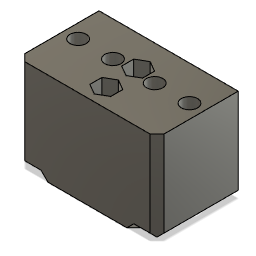
Hanger__Ceiling__Interchange (Autodesk Fusion 360 design; units mm, degrees)
Autodesk Fusion 360 part; units mm, degrees
sketch "Sketch1" plane through (0, 0, 0) normal (0, 1, 0) x (1, 0, 0)
  line L0 (0, 0) -> (60, 0)
  line L1 (60, 0) -> (60, -40)
  line L2 (60, -40) -> (0, -40)
  line L3 (0, -40) -> (0, 0)
  dimension "d1" = 60
  dimension "d2" = 40
  constraint horizontal L0
  constraint vertical L1
  constraint horizontal L2
  constraint vertical L3
  constraint coincident L0.start L3.end
  measures "d1" distance of L0.start L0.end
  measures "d2" distance of L0.start L2.end
extrude "Extrude1" add sketch "Sketch1" along normal blind 25
sketch "Sketch2" plane through (0, 25, 0) normal (0, 1, 0) x (-1, 0, 0)
  line L0 (0, 40) -> (-60, 40)
  line L1 (-60, 40) -> (-60, 0)
  line L2 (-60, 0) -> (0, 0)
  line L3 (0, 0) -> (0, 40)
  line L4 (-30, 0) -> (-30, 20)
  line L5 (-30, 20) -> (-39, 20)
  line L6 (-30, 20) -> (-21, 20)
  line L7 (-21, 20) -> (-6, 20)
  line L8 (-39, 20) -> (-54, 20)
  circle A0 centre (-21, 20) radius 3.5
  circle A1 centre (-39, 20) radius 3.5
  circle A2 centre (-54, 20) radius 3.5
  circle A3 centre (-6, 20) radius 3.5
  dimension "d5" = 20
  dimension "d6" = 9
  dimension "d7" = 9
  dimension "d8" = 15
  dimension "d9" = 15
  dimension "d10" = 7
  dimension "d11" = 7
  dimension "d12" = 7
  dimension "d13" = 7
  constraint midpoint L2 L4.start
  constraint perpendicular L0 L4
  constraint perpendicular L4 L5
  constraint perpendicular L4 L6
  constraint parallel L6 L7
  constraint perpendicular L4 L8
  constraint coincident L6.end L7.start
  constraint coincident L5.end L8.start
  constraint coincident L8.end A2.centre
  constraint coincident L7.end A3.centre
  measures "d5" distance of L4.start L4.end
  measures "d6" distance of L4.end L5.end
  measures "d7" distance of L4.end L6.end
  measures "d8" distance of L6.end L7.end
  measures "d9" distance of L5.end L8.end
  measures "d10" diameter of A0
  measures "d11" diameter of A1
  measures "d12" diameter of A2
  measures "d13" diameter of A3
extrude "Extrude2" cut sketch "Sketch2" against normal blind 25 contours L5 L8 A1 | L5 L8 A1 | L6 L7 A0 | L6 L7 A0 | A2 | A3
sketch "Sketch3" plane through (0, 0, 0) normal (0, -1, 0) x (1, 0, 0)
  circle A0 centre (21, 20) radius 3.5
  circle A1 centre (39, 20) radius 3.5
  circle A2 centre (6, 20) radius 3.5
  circle A3 centre (54, 20) radius 3.5
  line L0 (60, 40) -> (0, 40)
  line L1 (0, 40) -> (0, 0)
  line L2 (0, 0) -> (60, 0)
  line L3 (60, 0) -> (60, 40)
  circle A4 centre (6, 20) radius 6.5
  circle A5 centre (21, 20) radius 6.5
  circle A6 centre (39, 20) radius 6.5
  circle A7 centre (54, 20) radius 6.5
  dimension "d16" = 13
  dimension "d17" = 13
  dimension "d18" = 13
  dimension "d19" = 13
  constraint concentric A2 A4
  constraint concentric A0 A5
  constraint concentric A1 A6
  constraint concentric A3 A7
  measures "d16" diameter of A4
  measures "d17" diameter of A5
  measures "d18" diameter of A6
  measures "d19" diameter of A7
extrude "Extrude3" cut sketch "Sketch3" against normal blind 2 contours L3 A7 | L1 A4 | A5 | A6 picked at (59.1667, 20) picked at (0.8333, 20)
extrude "Extrude4" cut 4 faces at (0.8333, 2, 20) (26.4628, 2, 19.5032) (44.4758, 2, 19.6771) (59.1667, 2, 20) along direction (0, 1, 0) blind 13
sketch "Sketch4" plane through (0, 25, 0) normal (0, 1, 0) x (-1, 0, 0)
  circle A0 centre (-21, 20) radius 3.5
  circle A1 centre (-39, 20) radius 3.5
  circle A2 centre (-6, 20) radius 3.5
  circle A3 centre (-54, 20) radius 3.5
  line L0 (0, 40) -> (-60, 40)
  line L1 (-60, 40) -> (-60, 0)
  line L2 (-60, 0) -> (0, 0)
  line L3 (0, 0) -> (0, 40)
  line L4 (-30, 40) -> (-30, 0)
  line L5 (-30, 20) -> (-30, 26.85)
  line L6 (-30, 26.85) -> (-30, 13.15)
  circle A4 centre (-30, 13.15) radius 2
  circle A5 centre (-30, 26.85) radius 2
  dimension "d24" = 6.85
  dimension "d25" = 13.7
  dimension "d26" = 4
  dimension "d27" = 4
  constraint midpoint L0 L4.start
  constraint midpoint L2 L4.end
  constraint midpoint L4 L5.start
  constraint parallel L4 L5
  constraint parallel L4 L6
  constraint coincident L6.end A4.centre
  constraint coincident L5.end L6.start
  measures "d24" distance of L5.start L5.end
  measures "d25" distance of L5.end L6.end
  measures "d26" diameter of A4
  measures "d27" diameter of A5
sketch "Sketch5" plane through (0, 25, 0) normal (0, 1, 0) x (-1, 0, 0)
  circle A0 centre (-21, 20) radius 3.5
  circle A1 centre (-39, 20) radius 3.5
  circle A2 centre (-6, 20) radius 3.5
  circle A3 centre (-54, 20) radius 3.5
  line L0 (0, 40) -> (-60, 40)
  line L1 (-60, 40) -> (-60, 0)
  line L2 (-60, 0) -> (0, 0)
  line L3 (0, 0) -> (0, 40)
  line L4 (-34.5, 24.2519) -> (-30, 21.6538)
  line L5 (-30, 21.6538) -> (-25.5, 24.2519)
  line L6 (-25.5, 24.2519) -> (-25.5, 29.4481)
  line L7 (-25.5, 29.4481) -> (-30, 32.0462)
  line L8 (-30, 32.0462) -> (-34.5, 29.4481)
  line L9 (-34.5, 29.4481) -> (-34.5, 24.2519)
  line L10 (-34.5, 10.5519) -> (-30, 7.9538)
  line L11 (-30, 7.9538) -> (-25.5, 10.5519)
  line L12 (-25.5, 10.5519) -> (-25.5, 15.7481)
  line L13 (-25.5, 15.7481) -> (-30, 18.3462)
  line L14 (-30, 18.3462) -> (-34.5, 15.7481)
  line L15 (-34.5, 15.7481) -> (-34.5, 10.5519)
  point P0 (-30, 26.85)
  point P1 (-30, 13.15)
  dimension "d30" = 4.5
  dimension "d31" = 4.5
  measures "d30" distance of P0 L9
  measures "d31" distance of P1 L15
sketch "Sketch6" plane through (0, 0, 0) normal (0, -1, 0) x (1, 0, 0)
  arc A0 (60, 22.5) -> (60, 17.5) centre (54, 20) ccw
  line L0 (60, 22.5) -> (60, 40)
  line L1 (60, 40) -> (0, 40)
  line L2 (0, 40) -> (0, 22.5)
  arc A1 (0, 17.5) -> (0, 22.5) centre (6, 20) ccw
  line L3 (0, 17.5) -> (0, 0)
  line L4 (0, 0) -> (60, 0)
  line L5 (60, 0) -> (60, 17.5)
  circle A2 centre (21, 20) radius 6.5
  circle A3 centre (39, 20) radius 6.5
  circle A4 centre (6, 20) radius 5
  circle A5 centre (21, 20) radius 5
  circle A6 centre (54, 20) radius 5
  circle A7 centre (39, 20) radius 5
  circle A8 centre (6, 20) radius 6.5
  circle A9 centre (54, 20) radius 6.5
  circle A10 centre (39, 20) radius 6.5
  circle A11 centre (21, 20) radius 6.5
  dimension "d32" = 10
  dimension "d33" = 10
  dimension "d34" = 10
  dimension "d35" = 10
  constraint concentric A1 A4
  constraint concentric A2 A5
  constraint concentric A0 A6
  constraint concentric A3 A7
  constraint concentric A4 A8
  constraint concentric A6 A9
  constraint concentric A7 A10
  constraint concentric A5 A11
  measures "d32" diameter of A4
  measures "d33" diameter of A5
  measures "d34" diameter of A6
  measures "d35" diameter of A7
extrude "Extrude6" add sketch "Sketch6" against normal blind 15 contours A0 A9 | A1 A8 | A2 A11 | A3 A10
sketch "Sketch7" plane through (0, 25, 0) normal (0, 1, 0) x (-1, 0, 0)
  circle A0 centre (-21, 20) radius 3.5
  circle A1 centre (-39, 20) radius 3.5
  circle A2 centre (-6, 20) radius 3.5
  circle A3 centre (-54, 20) radius 3.5
  line L0 (0, 40) -> (-60, 40)
  line L1 (-60, 40) -> (-60, 0)
  line L2 (-60, 0) -> (0, 0)
  line L3 (0, 0) -> (0, 40)
  line L4 (-60, 40) -> (0, 40)
  line L5 (0, 40) -> (0, 0)
  line L6 (0, 0) -> (-60, 0)
  line L7 (-60, 0) -> (-60, 40)
  line L8 (-63.5098, 43.7878) -> (2.9374, 43.7878)
  line L9 (2.9374, 43.7878) -> (2.9374, -3.4155)
  line L10 (2.9374, -3.4155) -> (-63.5098, -3.4155)
  line L11 (-63.5098, -3.4155) -> (-63.5098, 43.7878)
  constraint horizontal L4
  constraint vertical L5
  constraint horizontal L6
  constraint vertical L7
  constraint coincident L2.end L3.start
  constraint coincident L0.end L1.start
  constraint horizontal L8
  constraint vertical L9
  constraint horizontal L10
  constraint vertical L11
extrude "Extrude8" cut sketch "Sketch7" against normal blind 41 contours L8 L9 L10 L11
sketch "Sketch8" plane through (0, 0, 0) normal (-1, 0, 0) x (0, 0, 1)
  line L0 (0, 0) -> (40, 0)
  line L1 (40, 0) -> (40, 25)
  line L2 (40, 25) -> (0, 25)
  line L3 (0, 25) -> (0, 0)
  line L4 (40, 0) -> (37, 0)
  line L5 (40, 0) -> (40, 3)
  line L6 (40, 3) -> (37, 0)
  dimension "d42" = 3
  dimension "d43" = 3
  constraint coincident L0.end L1.start
  constraint perpendicular L1 L4
  constraint perpendicular L0 L5
  measures "d42" distance of L0.end L4.end
  measures "d43" distance of L0.end L5.end
extrude "Extrude9" cut sketch "Sketch8" against normal blind 10 contours L0 L1 L4 L5 L6
extrude "Extrude10" cut 1 faces at (10, 1, 39) along direction (-1, 0, 0) blind -40 and the other way blind 50
sketch "Sketch9" plane through (0, 25, 0) normal (0, 1, 0) x (-1, 0, 0)
  circle A0 centre (-21, 20) radius 3.5
  circle A1 centre (-39, 20) radius 3.5
  circle A2 centre (-6, 20) radius 3.5
  circle A3 centre (-54, 20) radius 3.5
  line L0 (0, 40) -> (-60, 40)
  line L1 (-60, 40) -> (-60, 0)
  line L2 (-60, 0) -> (0, 0)
  line L3 (0, 0) -> (0, 40)
  line L4 (-30, 40) -> (-30, 31.85)
  circle A4 centre (-30, 31.85) radius 2
  line L5 (-30, 31.85) -> (-30, 18.15)
  circle A5 centre (-30, 18.15) radius 2
  dimension "d50" = 8.15
  dimension "d51" = 4
  dimension "d52" = 13.7
  dimension "d53" = 4
  constraint midpoint L0 L4.start
  constraint perpendicular L0 L4
  constraint coincident L4.end A4.centre
  constraint parallel L4 L5
  constraint coincident L5.end A5.centre
  measures "d50" distance of L4.start L4.end
  measures "d51" diameter of A4
  measures "d52" distance of L4.end L5.end
  measures "d53" diameter of A5
extrude "Extrude11" cut sketch "Sketch9" against normal blind 25 contours L4 A4 L5 | L4 A4 L5 | A5
sketch "Sketch10" plane through (0, 25, 0) normal (0, 1, 0) x (-1, 0, 0)
  circle A0 centre (-30, 31.85) radius 2
  circle A1 centre (-30, 18.15) radius 2
  circle A2 centre (-21, 20) radius 3.5
  circle A3 centre (-39, 20) radius 3.5
  circle A4 centre (-6, 20) radius 3.5
  circle A5 centre (-54, 20) radius 3.5
  line L0 (0, 40) -> (-60, 40)
  line L1 (-60, 40) -> (-60, 0)
  line L2 (-60, 0) -> (0, 0)
  line L3 (0, 0) -> (0, 40)
  line L4 (-34.5, 29.2519) -> (-30, 26.6538)
  line L5 (-30, 26.6538) -> (-25.5, 29.2519)
  line L6 (-25.5, 29.2519) -> (-25.5, 34.4481)
  line L7 (-25.5, 34.4481) -> (-30, 37.0462)
  line L8 (-30, 37.0462) -> (-34.5, 34.4481)
  line L9 (-34.5, 34.4481) -> (-34.5, 29.2519)
  line L10 (-34.5, 15.5519) -> (-30, 12.9538)
  line L11 (-30, 12.9538) -> (-25.5, 15.5519)
  line L12 (-25.5, 15.5519) -> (-25.5, 20.7481)
  line L13 (-25.5, 20.7481) -> (-30, 23.3462)
  line L14 (-30, 23.3462) -> (-34.5, 20.7481)
  line L15 (-34.5, 20.7481) -> (-34.5, 15.5519)
  point P0 (-30, 31.85)
  point P1 (-30, 18.15)
  dimension "d56" = 4.5
  dimension "d57" = 4.5
  constraint coincident P0 A0.centre
  constraint coincident P1 A1.centre
  measures "d56" distance of P0 L9
  measures "d57" distance of P1 L15
extrude "Extrude12" cut sketch "Sketch10" against normal blind 15 contours L4 L5 L6 L7 L8 L9 | L10 L11 L12 L13 L14 L15
sketch "Sketch11" plane through (0, 0, 0) normal (0, -1, 0) x (1, 0, 0)
sketch "Sketch12" plane through (0, 0, 40) normal (0, 0, 1) x (1, 0, 0)
sketch "Sketch13" plane through (0, 0, 0) normal (0, -1, 0) x (1, 0, 0)
sketch "Sketch14" plane through (0, 0, 40) normal (0, 0, 1) x (1, 0, 0)
ref_plane "WorkPlane1" through (11.5, 0, 38.5) normal (-0.579228, -0.573576, 0.579228) x (-0.707107, 0, -0.707107)
sketch "Sketch15" plane through (11.5, 0, 38.5) normal (-0.579228, -0.573576, 0.579228) x (-0.707107, 0, -0.707107)
  line L0 (2.1213, 0, 0) -> (0, -3.6742, 0.017)
  line L1 (0, -3.6742, 0.017) -> (-2.1213, 0, 0)
  line L2 (-2.1213, 0) -> (2.1213, 0)
  point P0 (2.1213, 0)
  point P1 (0, -3.6742)
  point P2 (-2.1213, 0)
  constraint coincident P0 L2.end
  constraint coincident P2 L2.start
extrude "Extrude13" cut sketch "Sketch15" along normal blind 5 contours L0 L1 L2 in plane through (11.5, 0, 38.5) normal (-0.57735, -0.57735, 0.57735)
ref_plane "WorkPlane2" through (48.5, 1.5, 40) normal (0.579228, -0.579228, 0.573576) x (0.707107, 0.707107, 0)
sketch "Sketch16" plane through (48.5, 1.5, 40) normal (0.579228, -0.579228, 0.573576) x (0.707107, 0.707107, 0)
  line L0 (-2.1213, 0) -> (2.1213, 0)
  line L1 (2.1213, 0, 0) -> (0, -3.6742, 0.017)
  line L2 (0, -3.6742, 0.017) -> (-2.1213, 0, 0)
  point P0 (-2.1213, 0)
  point P1 (2.1213, 0)
  point P2 (0, -3.6742)
  constraint coincident P0 L0.start
  constraint coincident P1 L0.end
extrude "Extrude14" cut sketch "Sketch16" along normal blind 5 contours L0 L1 L2 in plane through (48.5, 1.5, 40) normal (0.57735, -0.57735, 0.57735)
chamfer "Chamfer1" distance 3 distance2 3 2 edges at (0, 14, 40) (60, 14, 40) measured on face at (0, 16.6667, 25.6667) measured on face at (23.3333, 17.6667, 40)
chamfer "Chamfer2" distance 3 angle 45 1 edges at (60, 0, 18.5)
chamfer "Chamfer3" distance 3 angle 45 1 edges at (0, 0, 18.5)
extrude "Extrude15" add 1 faces at (30, 25, 4.3179) along direction (0, 1, 0) blind 15
extrude "Extrude16" add 2 faces at (28.1667, 10, 28.6746) (28.1667, 10, 14.9746) along direction (0, 1, 0) blind 15
extrude "Extrude17" cut 4 faces at (10.4684, 15, 19.5777) (25.1536, 15, 19.349) (34.8464, 15, 19.349) (58.4684, 15, 19.5777) along direction (0, 1, 0) blind 15
extrude "Extrude18" cut 1 faces at (39, 26.6667, 0) along direction (0, 0, 1) blind 5
